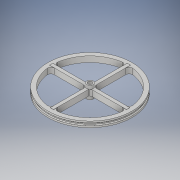
# Autodesk Inventor part: MTV Wheel (10.15)
Saved by Autodesk Inventor 2018 (Build 220112000, 112)
## iProperties
Created: 2018-10-16
Part Number: MTV Wheel (10.15)
Material: Generic
Document SubType Name: Modeling
Designer: Aditya Kendre
Density: 1 g/cm^3
Appearance: Default
Author: Aditya Kendre
## iProperties of the stored document MTV Wheel (10_3DPrint.ipt
Created: 2018-10-16
Part Number: MTV Wheel (10_3DPrint
Material: Generic
Document SubType Name: Modeling
Designer: Aditya Kendre
Density: 1 g/cm^3
Appearance: Default
Author: Aditya Kendre
Autodesk Inventor part; units mm, degrees
ref_plane "YZ Plane" through (0, 0, 0) normal (1, 0, 0) x (0, 1, 0)
ref_plane "XZ Plane" through (0, 0, 0) normal (0, 1, 0) x (-1, 0, 0)
ref_plane "XY Plane" through (0, 0, 0) normal (0, 0, 1) x (1, 0, 0)
sketch "Sketch1" plane through (0, 0, 0) normal (0, 1, 0) x (-1, 0, 0)
  circle A0 centre (0, 0) radius 39.6875
  dimension "d0" = 79.375
  constraints: 1 centre point, 1 coincident
  measures "d0" diameter of A0
extrude "Extrusion1" add sketch "Sketch1" along normal blind 2.3813
sketch "Sketch2" plane through (0, 2.3813, 0) normal (0, 1, 0) x (1, 0, 0)
  circle A0 centre (0, 0) radius 40.4876
  dimension "d3" = 80.9752
  constraints: 1 centre point, 1 coincident
  measures "d3" diameter of A0
sketch "Sketch3" plane through (0, 0, 0) normal (0, -1, 0) x (1, 0, 0)
  point P0 (0, 0)
extrude "Extrusion2" add sketch "Sketch2" along normal blind 1.5875
sketch "Sketch4" plane through (0, 0, 0) normal (0, -1, 0) x (1, 0, 0)
  circle A0 centre (0, 0) radius 40.4876
  dimension "d6" = 80.9752
  constraints: 1 centre point, 1 coincident
  measures "d6" diameter of A0
extrude "Extrusion3" add sketch "Sketch4" along normal blind 1.5875
fillet "Fillet1" radius 0.762 2 edges at (39.6875, 0, 0) (39.6875, 2.3813, 0)
sketch "Sketch5" plane through (0, 3.9688, 0) normal (0, 1, 0) x (1, 0, 0)
  circle A0 centre (0, 0) radius 36.5125
  dimension "d10" = 73.025
  constraints: 1 centre point, 1 coincident
  measures "d10" diameter of A0
extrude "Extrusion4" cut sketch "Sketch5" against normal blind 6.35
sketch "Sketch6" plane through (0, -1.5875, 0) normal (0, -1, 0) x (1, 0, 0)
  line L0 (36.703, 1.5875) -> (-37.4267, 1.5875)
  line L1 (-37.4267, 1.5875) -> (-37.4267, -1.5875)
  line L2 (-37.4267, -1.5875) -> (36.703, -1.5875)
  line L3 (36.703, -1.5875) -> (36.703, 1.5875)
  point P0 (0, 0)
  dimension "d13" = 3.175
  constraints: 8 end point, 2 parallel, 1 horizontal, 1 perpendicular
  measures "d13" distance of L1.end L0.end
extrude "Extrusion5" add sketch "Sketch6" against normal blind 5.715
sketch "Sketch7" plane through (0, -1.5875, 0) normal (0, -1, 0) x (1, 0, 0)
  line L0 (1.5875, 36.703) -> (-1.5875, 36.703)
  line L1 (-1.5875, 36.703) -> (-1.5875, -37.5002)
  line L2 (-1.5875, -37.5002) -> (1.5875, -37.5002)
  line L3 (1.5875, -37.5002) -> (1.5875, 36.703)
  point P0 (0, 0)
  dimension "d16" = 3.175
  constraints: 8 end point, 2 parallel, 1 horizontal, 1 perpendicular
  measures "d16" distance of L2.end L1.end
extrude "Extrusion6" add sketch "Sketch7" against normal blind 5.715
fillet "Fillet2" radius 3.175 1 edges at (36.478, 1.1906, 1.5875)
fillet "Fillet3" radius 3.175 1 edges at (36.478, 1.1906, -1.5875)
fillet "Fillet4" radius 3.175 6 edges at (1.5875, 1.1906, 36.478) (-36.478, 1.1906, -1.5875) (-1.5875, 1.1906, 36.478) (1.5875, 1.1906, -36.478) (-36.478, 1.1906, 1.5875) (-1.5875, 1.1906, -36.478)
sketch "Sketch8" plane through (0, -1.5875, 0) normal (0, -1, 0) x (1, 0, 0)
  circle A0 centre (0, 0) radius 3.175
  dimension "d22" = 6.35
  constraints: 1 centre point, 1 coincident
  measures "d22" diameter of A0
extrude "Extrusion7" add sketch "Sketch8" against normal blind 5.715
sketch "Sketch9" plane through (0, 4.1275, 0) normal (0, 1, 0) x (1, 0, 0)
  circle A0 centre (0, 0) radius 1.9939
  dimension "d25" = 3.9878
  constraints: 1 centre point, 1 coincident
  measures "d25" diameter of A0
extrude "Extrusion8" cut sketch "Sketch9" against normal blind 5.715
sketch "Sketch10" plane through (0, 4.1275, 0) normal (0, 1, 0) x (1, 0, 0)
  circle A0 centre (0, 0) radius 1.9939
  circle A1 centre (0, 0) radius 3.175
  constraints: 2 centre point, 2 coincident
extrude "Extrusion9" add sketch "Sketch10" along normal blind 3.175 and the other way blind 8.89
fillet "Fillet5" radius 3.175 7 edges at (2.7496, 1.27, -1.5875) (1.5875, 1.27, -2.7496) (-1.5875, 1.27, -2.7496) (-2.7496, 1.27, -1.5875) (-1.5875, 1.27, 2.7496) (-2.7496, 1.27, 1.5875) (2.7496, 1.27, 1.5875)
body "Solid1"
